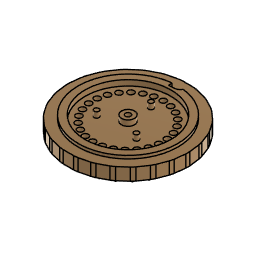
筐体 (Autodesk Fusion 360 archive; units mm, degrees)
design "ローターA"
Autodesk Fusion 360 part; units mm, degrees
sketch "スケッチ2" plane through (0, 0, 0) normal (0, 0, 1) x (1, 0, 0) in component "ローターA"
  circle A0 centre (0, 0) radius 23 construction
  circle A1 centre (0, 23) radius 2
  circle A2 centre (-5.5043, 22.3317) radius 2
  circle A3 centre (-10.6886, 20.3655) radius 2
  circle A4 centre (-15.2518, 17.2157) radius 2
  circle A5 centre (-18.9286, 13.0655) radius 2
  circle A6 centre (-21.5054, 8.1559) radius 2
  circle A7 centre (-22.8323, 2.7723) radius 2
  circle A8 centre (-22.8323, -2.7723) radius 2
  circle A9 centre (-21.5054, -8.1559) radius 2
  circle A10 centre (-18.9286, -13.0655) radius 2
  circle A11 centre (-15.2518, -17.2157) radius 2
  circle A12 centre (-10.6886, -20.3655) radius 2
  circle A13 centre (-5.5043, -22.3317) radius 2
  circle A14 centre (0, -23) radius 2
  circle A15 centre (5.5043, -22.3317) radius 2
  circle A16 centre (10.6886, -20.3655) radius 2
  circle A17 centre (15.2518, -17.2157) radius 2
  circle A18 centre (18.9286, -13.0655) radius 2
  circle A19 centre (21.5054, -8.1559) radius 2
  circle A20 centre (22.8323, -2.7723) radius 2
  circle A21 centre (22.8323, 2.7723) radius 2
  circle A22 centre (21.5054, 8.1559) radius 2
  circle A23 centre (18.9286, 13.0655) radius 2
  circle A24 centre (15.2518, 17.2157) radius 2
  circle A25 centre (10.6886, 20.3655) radius 2
  circle A26 centre (5.5043, 22.3317) radius 2
  circle A27 centre (0, 0) radius 4.25
  circle A28 centre (0, 0) radius 1.75
  circle A29 centre (0, 0) radius 28
  circle A30 centre (0, 0) radius 39
  line L0 (0, 0) -> (3.3913, -38.8523)
  line L1 (0, 0) -> (-3.3913, -38.8523)
  line L2 (3.3913, -38.8523) -> (-3.3913, -38.8523)
  line L3 (12.5907, -36.9117) -> (6.0052, -38.5349)
  line L4 (21.0584, -32.826) -> (15.0527, -35.978)
  line L5 (28.3022, -26.8325) -> (23.2254, -31.3302)
  line L6 (33.9013, -19.2796) -> (30.0483, -24.8616)
  line L7 (37.5301, -10.6063) -> (35.1249, -16.9481)
  line L8 (38.9778, -1.3165) -> (38.1602, -8.0497)
  line L9 (38.1602, 8.0497) -> (38.9778, 1.3165)
  line L10 (35.1249, 16.9481) -> (37.5301, 10.6063)
  line L11 (30.0483, 24.8616) -> (33.9013, 19.2796)
  line L12 (23.2254, 31.3302) -> (28.3022, 26.8325)
  line L13 (15.0527, 35.978) -> (21.0584, 32.826)
  line L14 (6.0052, 38.5349) -> (12.5907, 36.9117)
  line L15 (-3.3913, 38.8523) -> (3.3913, 38.8523)
  line L16 (-12.5907, 36.9117) -> (-6.0052, 38.5349)
  line L17 (-21.0584, 32.826) -> (-15.0527, 35.978)
  line L18 (-28.3022, 26.8325) -> (-23.2254, 31.3302)
  line L19 (-33.9013, 19.2796) -> (-30.0483, 24.8616)
  line L20 (-37.5301, 10.6063) -> (-35.1249, 16.9481)
  line L21 (-38.9778, 1.3165) -> (-38.1602, 8.0497)
  line L22 (-38.1602, -8.0497) -> (-38.9778, -1.3165)
  line L23 (-35.1249, -16.9481) -> (-37.5301, -10.6063)
  line L24 (-30.0483, -24.8616) -> (-33.9013, -19.2796)
  line L25 (-23.2254, -31.3302) -> (-28.3022, -26.8325)
  line L26 (-15.0527, -35.978) -> (-21.0584, -32.826)
  line L27 (-6.0052, -38.5349) -> (-12.5907, -36.9117)
  dimension "d10" = 46
  dimension "d11" = 4
  dimension "d13" = 360
  dimension "d24" = 8.5
  dimension "d37" = 3.5
  dimension "d64" = 56
  dimension "d65" = 78
  dimension "d67" = 360
  constraint coincident A0.centre A27.centre
  constraint coincident A0 A1.centre
  constraint concentric A0 A27
  constraint concentric A0 A28
  constraint concentric A0 A29
  constraint coincident A30 L0.end
  constraint coincident A30 L1.end
  constraint tangent A14 L0
  constraint tangent A14 L1
  measures "d10" diameter of A0
  measures "d11" diameter of A1
  measures "d24" diameter of A27
  measures "d37" diameter of A28
  measures "d64" diameter of A29
  measures "d65" diameter of A30
extrude "押し出し4" add sketch "スケッチ2" along normal blind 2 contours A14 A29 L0 L1 | A14 A27 L0 L1 | A27 A29 L0 L1 makes body 1 in component "ローターA"
sketch "スケッチ4" plane through (0, 0, 2) normal (0, 0, 1) x (-1, 0, 0) in component "ローターA"
  circle A0 centre (0, 0) radius 15 construction
  circle A1 centre (0, -15) radius 1.6
  circle A2 centre (12.9904, 7.5) radius 1.6
  circle A3 centre (-12.9904, 7.5) radius 1.6
  circle A4 centre (0, 0) radius 4.25
  circle A5 centre (-18.9286, -13.0655) radius 2
  circle A6 centre (-5.5043, -22.3317) radius 2
  circle A7 centre (-21.5054, -8.1559) radius 2
  circle A8 centre (15.2518, 17.2157) radius 2
  circle A9 centre (-10.6886, 20.3655) radius 2
  circle A10 centre (18.9286, 13.0655) radius 2
  circle A11 centre (10.6886, -20.3655) radius 2
  circle A12 centre (-15.2518, -17.2157) radius 2
  circle A13 centre (18.9286, -13.0655) radius 2
  circle A14 centre (-22.8323, 2.7723) radius 2
  circle A15 centre (-10.6886, -20.3655) radius 2
  circle A16 centre (-22.8323, -2.7723) radius 2
  circle A17 centre (21.5054, 8.1559) radius 2
  circle A18 centre (22.8323, -2.7723) radius 2
  circle A19 centre (15.2518, -17.2157) radius 2
  circle A20 centre (0, -23) radius 2
  circle A21 centre (22.8323, 2.7723) radius 2
  circle A22 centre (-5.5043, 22.3317) radius 2
  circle A23 centre (-18.9286, 13.0655) radius 2
  circle A24 centre (10.6886, 20.3655) radius 2
  circle A25 centre (-15.2518, 17.2157) radius 2
  circle A26 centre (-21.5054, 8.1559) radius 2
  circle A27 centre (5.5043, -22.3317) radius 2
  circle A28 centre (21.5054, -8.1559) radius 2
  circle A29 centre (5.5043, 22.3317) radius 2
  circle A30 centre (0, 23) radius 2
  circle A31 centre (0, 0) radius 28
  dimension "d31" = 30
  dimension "d32" = 3.2
  dimension "d16" = 3.2
  dimension "d17" = 3.2
  constraint coincident A0.centre A4.centre
  constraint coincident A0 A1.centre
  measures "d31" diameter of A0
  measures "d32" diameter of A1
  measures "d16" diameter of A3
  measures "d17" diameter of A2
extrude "押し出し8" add sketch "スケッチ4" along normal blind 8 contours A1 | A2 | A3 bodies 1 in component "ローターA"
extrude "押し出し9" add sketch "スケッチ2" along normal blind 10 contours A27 A28 L0 L1 | A27 A28 L0 L1 bodies 1 in component "ローターA"
extrude "押し出し13" add sketch "スケッチ2" along normal blind 8 contours A29 L0 L1 L2 | A29 A30 L0 L1 L3 L4 L5 L6 L7 L8 L9 L10 L11 L12 L13 L14 L15 L16 L17 L18 L19 L20 L21 L22 L23 L24 L25 L26 L27 bodies 1 in component "ローターA"
sketch "スケッチ9" plane through (0, 0, 0) normal (0, 0, 1) x (1, 0, 0) in component "ローターA"
  circle A0 centre (0, 0) radius 28
  circle A1 centre (18.9286, -13.0655) radius 2
  circle A2 centre (21.5054, -8.1559) radius 2
  circle A3 centre (22.8323, 2.7723) radius 2
  circle A4 centre (22.8323, -2.7723) radius 2
  circle A5 centre (21.5054, 8.1559) radius 2
  circle A6 centre (18.9286, 13.0655) radius 2
  circle A7 centre (15.2518, 17.2157) radius 2
  circle A8 centre (10.6886, 20.3655) radius 2
  circle A9 centre (5.5043, 22.3317) radius 2
  circle A10 centre (0, 23) radius 2
  circle A11 centre (-5.5043, 22.3317) radius 2
  circle A12 centre (-10.6886, 20.3655) radius 2
  circle A13 centre (-15.2518, 17.2157) radius 2
  circle A14 centre (-18.9286, 13.0655) radius 2
  circle A15 centre (-21.5054, 8.1559) radius 2
  circle A16 centre (-22.8323, 2.7723) radius 2
  circle A17 centre (-22.8323, -2.7723) radius 2
  circle A18 centre (-21.5054, -8.1559) radius 2
  circle A19 centre (-18.9286, -13.0655) radius 2
  circle A20 centre (-15.2518, -17.2157) radius 2
  circle A21 centre (-10.6886, -20.3655) radius 2
  circle A22 centre (-5.5043, -22.3317) radius 2
  circle A23 centre (0, -23) radius 2
  circle A24 centre (5.5043, -22.3317) radius 2
  circle A25 centre (10.6886, -20.3655) radius 2
  circle A26 centre (15.2518, -17.2157) radius 2
  circle A27 centre (0, 0) radius 30 construction
  circle A28 centre (0, 0) radius 34 construction
  circle A29 centre (0, 0) radius 32.5
  line L0 (-3.3413, 29.8133) -> (0, 0) construction
  arc A30 (0, 30) -> (-3.3413, 29.8133) centre (0, 0) ccw
  arc A31 (0, 30) -> (3.6197, 32.2978) centre (0, 34) ccw
  line L1 (-3.3413, 29.8133) -> (-3.6197, 32.2978)
  line L2 (-10.379, 28.1474) -> (-11.2439, 30.493)
  arc A32 (-7.1795, 29.1283) -> (-10.379, 28.1474) centre (0, 0) ccw
  arc A33 (-7.1795, 29.1283) -> (-4.2148, 32.2255) centre (-8.1367, 33.012) ccw
  line L3 (-16.8135, 24.8456) -> (-18.2147, 26.9161)
  arc A34 (-13.9417, 26.5637) -> (-16.8135, 24.8456) centre (0, 0) ccw
  arc A35 (-13.9417, 26.5637) -> (-11.8044, 30.2805) centre (-15.8006, 30.1055) ccw
  line L4 (-22.2709, 20.0999) -> (-24.1268, 21.7749)
  arc A36 (-19.8937, 22.4553) -> (-22.2709, 20.0999) centre (0, 0) ccw
  arc A37 (-19.8937, 22.4553) -> (-18.708, 26.5756) centre (-22.5462, 25.4494) ccw
  line L5 (-26.434, 14.1861) -> (-28.6368, 15.3683)
  arc A38 (-24.6895, 17.0419) -> (-26.434, 14.1861) centre (0, 0) ccw
  arc A39 (-24.6895, 17.0419) -> (-24.5243, 21.3262) centre (-27.9815, 19.3142) ccw
  line L6 (-29.0608, 7.4478) -> (-31.4825, 8.0684)
  arc A40 (-28.0505, 10.6381) -> (-29.0608, 7.4478) centre (0, 0) ccw
  arc A41 (-28.0505, 10.6381) -> (-28.9154, 14.8375) centre (-31.7906, 12.0566) ccw
  line L7 (-29.9987, 0.2767) -> (-32.4986, 0.2997)
  arc A42 (-29.7813, 3.6161) -> (-29.9987, 0.2767) centre (0, 0) ccw
  arc A43 (-29.7813, 3.6161) -> (-31.626, 7.4864) centre (-33.7521, 4.0982) ccw
  line L8 (-29.1932, -6.9105) -> (-31.626, -7.4864)
  arc A44 (-29.7813, -3.6161) -> (-29.1932, -6.9105) centre (0, 0) ccw
  arc A45 (-29.7813, -3.6161) -> (-32.4986, -0.2997) centre (-33.7521, -4.0982) ccw
  line L9 (-26.6911, -13.6961) -> (-28.9154, -14.8375)
  arc A46 (-28.0505, -10.6381) -> (-26.6911, -13.6961) centre (0, 0) ccw
  arc A47 (-28.0505, -10.6381) -> (-31.4825, -8.0684) centre (-31.7906, -12.0566) ccw
  line L10 (-22.6378, -19.6857) -> (-24.5243, -21.3262)
  arc A48 (-24.6895, -17.0419) -> (-22.6378, -19.6857) centre (0, 0) ccw
  arc A49 (-24.6895, -17.0419) -> (-28.6368, -15.3683) centre (-27.9815, -19.3142) ccw
  line L11 (-17.2689, -24.5313) -> (-18.708, -26.5756)
  arc A50 (-19.8937, -22.4553) -> (-17.2689, -24.5313) centre (0, 0) ccw
  arc A51 (-19.8937, -22.4553) -> (-24.1268, -21.7749) centre (-22.5462, -25.4494) ccw
  line L12 (-10.8964, -27.9512) -> (-11.8044, -30.2805)
  arc A52 (-13.9417, -26.5637) -> (-10.8964, -27.9512) centre (0, 0) ccw
  arc A53 (-13.9417, -26.5637) -> (-18.2147, -26.9161) centre (-15.8006, -30.1055) ccw
  line L13 (-3.8906, -29.7467) -> (-4.2148, -32.2255)
  arc A54 (-7.1795, -29.1283) -> (-3.8906, -29.7467) centre (0, 0) ccw
  arc A55 (-7.1795, -29.1283) -> (-11.2439, -30.493) centre (-8.1367, -33.012) ccw
  line L14 (3.3413, -29.8133) -> (3.6197, -32.2978)
  arc A56 (0, -30) -> (3.3413, -29.8133) centre (0, 0) ccw
  arc A57 (0, -30) -> (-3.6197, -32.2978) centre (0, -34) ccw
  line L15 (10.379, -28.1474) -> (11.2439, -30.493)
  arc A58 (7.1795, -29.1283) -> (10.379, -28.1474) centre (0, 0) ccw
  arc A59 (7.1795, -29.1283) -> (4.2148, -32.2255) centre (8.1367, -33.012) ccw
  line L16 (16.8135, -24.8456) -> (18.2147, -26.9161)
  arc A60 (13.9417, -26.5637) -> (16.8135, -24.8456) centre (0, 0) ccw
  arc A61 (13.9417, -26.5637) -> (11.8044, -30.2805) centre (15.8006, -30.1055) ccw
  line L17 (22.2709, -20.0999) -> (24.1268, -21.7749)
  arc A62 (19.8937, -22.4553) -> (22.2709, -20.0999) centre (0, 0) ccw
  arc A63 (19.8937, -22.4553) -> (18.708, -26.5756) centre (22.5462, -25.4494) ccw
  line L18 (26.434, -14.1861) -> (28.6368, -15.3683)
  arc A64 (24.6895, -17.0419) -> (26.434, -14.1861) centre (0, 0) ccw
  arc A65 (24.6895, -17.0419) -> (24.5243, -21.3262) centre (27.9815, -19.3142) ccw
  line L19 (29.0608, -7.4478) -> (31.4825, -8.0684)
  arc A66 (28.0505, -10.6381) -> (29.0608, -7.4478) centre (0, 0) ccw
  arc A67 (28.0505, -10.6381) -> (28.9154, -14.8375) centre (31.7906, -12.0566) ccw
  line L20 (29.9987, -0.2767) -> (32.4986, -0.2997)
  arc A68 (29.7813, -3.6161) -> (29.9987, -0.2767) centre (0, 0) ccw
  arc A69 (29.7813, -3.6161) -> (31.626, -7.4864) centre (33.7521, -4.0982) ccw
  line L21 (29.1932, 6.9105) -> (31.626, 7.4864)
  arc A70 (29.7813, 3.6161) -> (29.1932, 6.9105) centre (0, 0) ccw
  arc A71 (29.7813, 3.6161) -> (32.4986, 0.2997) centre (33.7521, 4.0982) ccw
  line L22 (26.6911, 13.6961) -> (28.9154, 14.8375)
  arc A72 (28.0505, 10.6381) -> (26.6911, 13.6961) centre (0, 0) ccw
  arc A73 (28.0505, 10.6381) -> (31.4825, 8.0684) centre (31.7906, 12.0566) ccw
  line L23 (22.6378, 19.6857) -> (24.5243, 21.3262)
  arc A74 (24.6895, 17.0419) -> (22.6378, 19.6857) centre (0, 0) ccw
  arc A75 (24.6895, 17.0419) -> (28.6368, 15.3683) centre (27.9815, 19.3142) ccw
  line L24 (17.2689, 24.5313) -> (18.708, 26.5756)
  arc A76 (19.8937, 22.4553) -> (17.2689, 24.5313) centre (0, 0) ccw
  arc A77 (19.8937, 22.4553) -> (24.1268, 21.7749) centre (22.5462, 25.4494) ccw
  line L25 (10.8964, 27.9512) -> (11.8044, 30.2805)
  arc A78 (13.9417, 26.5637) -> (10.8964, 27.9512) centre (0, 0) ccw
  arc A79 (13.9417, 26.5637) -> (18.2147, 26.9161) centre (15.8006, 30.1055) ccw
  line L26 (3.8906, 29.7467) -> (4.2148, 32.2255)
  arc A80 (7.1795, 29.1283) -> (3.8906, 29.7467) centre (0, 0) ccw
  arc A81 (7.1795, 29.1283) -> (11.2439, 30.493) centre (8.1367, 33.012) ccw
  circle A82 centre (0, 0) radius 1.75
  circle A83 centre (0, 0) radius 4.25
  circle A84 centre (0, 0) radius 18
  dimension "d70" = 56
  dimension "d71" = 60
  dimension "d72" = 68
  dimension "d73" = 65
  dimension "d74" = 4
  dimension "d76" = 360
  dimension "d79" = 36
  constraint coincident A28 A31.centre
  constraint tangent A27 A31
  constraint concentric A0 A29
  constraint coincident A0.centre A27.centre
  constraint coincident A27 A30.start
  constraint coincident A29 A31.end
  constraint coincident A29 L1.end
  constraint collinear L0 L1
  constraint concentric A76 A84
  measures "d70" diameter of A0
  measures "d71" diameter of A27
  measures "d72" diameter of A28
  measures "d73" diameter of A29
  measures "d74" radius of A31
  measures "d79" diameter of A84
extrude "押し出し14" add sketch "スケッチ9" against normal blind 5 contours A0 | A29 A30 A31 L1 L2 A32 A33 L3 A34 A35 L4 A36 A37 L5 A38 A39 L6 A40 A41 L7 A42 A43 L8 A44 A45 L9 A46 A47 L10 A48 A49 L11 A50 A51 L12 A52 A53 L13 A54 A55 L14 A56 A57 L15 A58 A59 L16 A60 A61 L17 A62 A63 L18 A64 A65 L19 A66 A67 L20 A68 A69 L21 A70 A71 L22 A72 A73 L23 A74 A75 L24 A76 A77 L25 A78 A79 L26 A80 A81 | A83 bodies 1 in component "ローターA"
copy_body "ボディ -> コンポーネント2" bodies 1 removing the originals makes body 2 in component "ローターA (1)"
extrude "押し出し1" add 1 faces at (-6.1521, -10.8292, 2) along direction (0, 0, 1) blind 4.4 on bodies 2 bodies 2 in component "ローターA (1)"
sketch "スケッチ1" plane through (0, 0, 8) normal (0, 0, 1) x (-1, 0, 0)
  arc A0 (0, -30) -> (-3.6197, -32.2978) centre (0, -34) ccw
  line L0 (3.3413, -29.8133) -> (3.6197, -32.2978)
  arc A1 (0, -30) -> (3.3413, -29.8133) centre (0, 0) ccw
  circle A2 centre (0, 0) radius 32.5
  circle A3 centre (0, 0) radius 28
  dimension "d9" = 56
  constraint concentric A2 A3
  measures "d9" diameter of A3
extrude "押し出し2" add sketch "スケッチ1" along normal blind 2 contours A0 L0 A1 A2 picked at (-5.9767, -30.17) bodies 2 in component "ローターA (1)"
component "ローターA" placed x (1, 0, 0) y (0, 1, 0) z (0, 0, 1) at (0, 0, 0)
component "ローターA (1)" placed x (1, 0, 0) y (0, 1, 0) z (0, 0, 1) at (0, 0, 0) in component "ローターA"
equation "d10 = ( 23 * 2 ) * 1 mm"
equation "d68 = 2.00 mm + 6 mm"
equation "d71 = d70 + 4 mm"
equation "d72 = d71 + 8 mm"
equation "d73 = d72 - 3 mm"
equation "d80 = 6.00 mm - 1.6 mm"

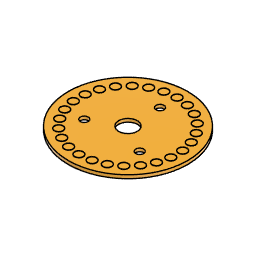
design "ローター基盤"
Autodesk Fusion 360 part; units mm, degrees
sketch "スケッチ1" plane through (0, 0, 0) normal (0, 0, 1) x (1, 0, 0)
  circle A0 centre (0, 0) radius 28
  circle A1 centre (0, 0) radius 23 construction
  circle A2 centre (0, 23) radius 2
  circle A3 centre (-5.5043, 22.3317) radius 2
  circle A4 centre (-10.6886, 20.3655) radius 2
  circle A5 centre (-15.2518, 17.2157) radius 2
  circle A6 centre (-18.9286, 13.0655) radius 2
  circle A7 centre (-21.5054, 8.1559) radius 2
  circle A8 centre (-22.8323, 2.7723) radius 2
  circle A9 centre (-22.8323, -2.7723) radius 2
  circle A10 centre (-21.5054, -8.1559) radius 2
  circle A11 centre (-18.9286, -13.0655) radius 2
  circle A12 centre (-15.2518, -17.2157) radius 2
  circle A13 centre (-10.6886, -20.3655) radius 2
  circle A14 centre (-5.5043, -22.3317) radius 2
  circle A15 centre (0, -23) radius 2
  circle A16 centre (5.5043, -22.3317) radius 2
  circle A17 centre (10.6886, -20.3655) radius 2
  circle A18 centre (15.2518, -17.2157) radius 2
  circle A19 centre (18.9286, -13.0655) radius 2
  circle A20 centre (21.5054, -8.1559) radius 2
  circle A21 centre (22.8323, -2.7723) radius 2
  circle A22 centre (22.8323, 2.7723) radius 2
  circle A23 centre (21.5054, 8.1559) radius 2
  circle A24 centre (18.9286, 13.0655) radius 2
  circle A25 centre (15.2518, 17.2157) radius 2
  circle A26 centre (10.6886, 20.3655) radius 2
  circle A27 centre (5.5043, 22.3317) radius 2
  dimension "d1" = 56
  dimension "d2" = 46
  dimension "d3" = 4
  dimension "d5" = 360
  constraint coincident A0.centre A1.centre
  constraint coincident A1 A2.centre
  measures "d1" diameter of A0
  measures "d2" diameter of A1
  measures "d3" diameter of A2
extrude "押し出し1" add sketch "スケッチ1" along normal blind 1.6 makes body 1
extrude "押し出し2" add sketch "スケッチ1" against normal blind 0.1 separate body contours A2 | A3 | A4 | A5 | A6 | A7 | A8 | A9 | A10 | A11 | A12 | A13 | A14 | A15 | A16 | A17 | A18 | A19 | A20 | A21 | A22 | A23 | A24 | A25 | A26 | A27 makes body 2 at (21.0897, -8.8759, 0) makes body 3 at (18.3138, 12.9661, 0) makes body 4 at (-11.0406, -19.27, 0) makes body 5 at (5.1709, 21.7543, 0) makes body 6 at (-5.4544, 21.7553, 0) makes body 7 at (-19.5435, -13.1649, 0) makes body 8 at (-23.248, -3.4923, 0) makes body 9 at (-23.4472, 2.673, 0) makes body 10 at (-10.0658, 19.9791, 0) makes body 11 at (15.8303, 17.2224, 0) makes body 12 at (15.7389, -18.4569, 0) makes body 13 at (0.0498, -23.5764, 0) makes body 14 at (22.2174, -2.8717, 0) makes body 15 at (21.0897, 7.436, 0) makes body 16 at (22.4166, 2.0524, 0) makes body 17 at (5.7478, -22.9522, 0) makes body 18 at (10.3367, 21.461, 0) makes body 19 at (-21.921, 7.436, 0) makes body 20 at (-15.4954, -16.5364, 0) makes body 21 at (-21.8165, -9.0291, 0) makes body 22 at (-19.3443, 12.3455, 0) makes body 23 at (-14.7631, 16.7623, 0) makes body 24 at (0.709, 23.5654, 0) makes body 25 at (18.513, -13.7854, 0) makes body 26 at (11.3115, -20.7519, 0) makes body 27 at (-5.2607, -22.9522, 0)
extrude "押し出し3" add sketch "スケッチ1" along normal blind 1.7 contours A2 | A3 | A4 | A5 | A6 | A7 | A8 | A9 | A10 | A11 | A12 | A13 | A14 | A15 | A16 | A17 | A18 | A19 | A20 | A21 | A22 | A23 | A24 | A25 | A26 | A27 bodies 1 2 3 4 5 6 7 8 9 10 11 12 13 14 15 16 17 18 19 20 21 22 23 24 25 26 27
sketch "スケッチ2" plane through (0, 0, 0) normal (0, 0, 1) x (1, 0, 0)
  circle A0 centre (0, 0) radius 15 construction
  circle A1 centre (0, 15) radius 2
  circle A2 centre (-12.9904, -7.5) radius 2
  circle A3 centre (12.9904, -7.5) radius 2
  circle A4 centre (0, 0) radius 4.5
  dimension "d12" = 30
  dimension "d13" = 4
  dimension "d15" = 360
  dimension "d16" = 9
  constraint coincident A0.centre A4.centre
  constraint coincident A0 A1.centre
  measures "d12" diameter of A0
  measures "d13" diameter of A1
  measures "d16" diameter of A4
extrude "押し出し4" cut sketch "スケッチ2" along normal up to surface (1.6 mm away) draft -5 bodies 1
copy_body "ボディ -> コンポーネント1" bodies 1 removing the originals makes body 28 in component "ローター基盤"
component "ローター基盤" placed x (1, 0, 0) y (0, 1, 0) z (0, 0, 1) at (0, 0, 0)
equation "d10 = 1.6 mm + 0.1 mm"

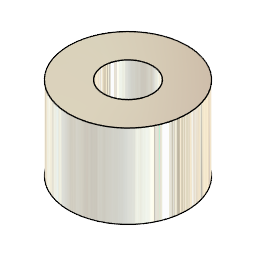
design "ロータースペーサー"
Autodesk Fusion 360 part; units mm, degrees
sketch "スケッチ1" plane through (0, 0, 0) normal (0, 0, 1) x (1, 0, 0)
  circle A0 centre (0, 0) radius 4.25
  circle A1 centre (0, 0) radius 1.75
  dimension "d1" = 3.5
  dimension "d2" = 8.5
  constraint coincident A0.centre A1.centre
  constraint concentric A0 A1
  measures "d1" diameter of A1
  measures "d2" diameter of A0
extrude "押し出し1" add sketch "スケッチ1" along normal blind 6 makes body 1
copy_body "ボディ -> コンポーネント1" bodies 1 removing the originals makes body 2 in component "ロータースペーサー"
component "ロータースペーサー" placed x (1, 0, 0) y (0, 1, 0) z (0, 0, 1) at (0, 0, 0)

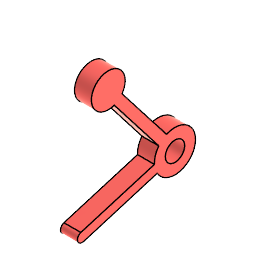
design "ラチェットストッパー"
Autodesk Fusion 360 part; units mm, degrees
sketch "スケッチ7" plane through (0, 0, 0) normal (1, 0, 0) x (0, 1, 0) in component "ラチェットストッパー 1"
  circle A0 centre (-13.9095, 17.7123) radius 3.5
  circle A1 centre (-0.1484, -0.0447) radius 2
  circle A2 centre (-0.1484, -0.0447) radius 2
  circle A3 centre (-0.1484, -0.0447) radius 4.25
  line L0 (-13.9095, 17.7123) -> (-0.1484, -0.0447) construction
  line L1 (-0.1129, -0.0906) -> (-13.9095, 17.7123) construction
  line L2 (-0.1484, -0.0447) -> (-19.2974, -5.8168) construction
  arc A4 (-19.5842, -4.8589) -> (-19.008, -6.7741) centre (-19.2974, -5.8168) ccw
  line L3 (-19.008, -6.7741) -> (-3.8251, -2.1765)
  line L4 (-0.1484, -0.0447) -> (-19.2974, -5.8168) construction
  line L5 (-1.8718, 0.4818) -> (-2.095, 0.4145)
  line L6 (-4.3918, -0.2818) -> (-19.5842, -4.8589)
  line L7 (-12.6841, 14.4338) -> (-3.4945, 2.5757)
  line L8 (-2.0168, 0.6689) -> (-1.8718, 0.4818)
  line L9 (-1.8847, 3.8344) -> (-11.0622, 15.6769)
  line L10 (-6.1824, -0.8212) -> (-5.6084, -2.7165)
  line L11 (-0.1484, -0.0447) -> (1.0781, -4.1139) construction
  dimension "d49" = 7
  dimension "d50" = 8.5
  dimension "d52" = 69
  dimension "d53" = 2
  dimension "d73" = 14
  dimension "d1" = 69
  dimension "d2" = 69
  dimension "d3" = 20
  constraint concentric A1 A2
  constraint concentric A2 A3
  constraint coincident A0.centre L0.start
  constraint coincident A1.centre A2.centre
  constraint parallel L0 L1
  constraint coincident L2.end A4.centre
  constraint parallel L2 L4
  constraint coincident A1 L5.end
  constraint coincident A3 L6.start
  constraint coincident A3 L7.end
  constraint coincident A1 L8.start
  constraint collinear L7 L8
  constraint coincident A3 L9.start
  constraint coincident A3 L3.end
  constraint coincident A0 L9.end
  constraint coincident A0 L7.start
  constraint coincident L6 L10.start
  constraint coincident L3 L10.end
  constraint perpendicular L3 L10
  constraint perpendicular L2 L11
  constraint coincident A3 L11.end
  measures "d49" diameter of A0
  measures "d50" diameter of A3
  measures "d52" angle of L1 L2
  measures "d53" diameter of A4
  measures "d73" distance of L2.end L10
  measures "d1" angle of L2 L7
  measures "d2" angle of L4 L9
  measures "d3" distance of A1.centre L2.end
extrude "押し出し1" add sketch "スケッチ7" along normal blind 3.5 in component "ラチェットストッパー"
component "ラチェットストッパー 1" placed x (1, 0, 0) y (0, 1, 0) z (0, 0, 1) at (0, 0, 0)
component "ラチェットストッパー" placed x (1, 0, 0) y (0, 1, 0) z (0, 0, 1) at (0, 0, 0) in component "ラチェットストッパー 1"
equation "d1 = d52"
equation "d2 = d52"

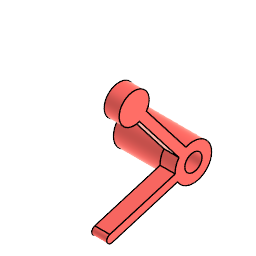
design "ラチェットストッパー&スペーサー"
Autodesk Fusion 360 part; units mm, degrees
sketch "スケッチ7" plane through (0, 0, 0) normal (1, 0, 0) x (0, 1, 0) in component "ラチェットストッパー 1"
  circle A0 centre (-13.9117, 17.7153) radius 3.5
  circle A1 centre (-0.1483, -0.0447) radius 2
  circle A2 centre (-0.1483, -0.0447) radius 2
  circle A3 centre (-0.1483, -0.0447) radius 4.25
  line L0 (-13.9117, 17.7153) -> (-0.1483, -0.0447) construction
  line L1 (-0.1124, -0.091) -> (-13.9117, 17.7153) construction
  line L2 (-0.1483, -0.0447) -> (-19.2973, -5.8168) construction
  arc A4 (-19.584, -4.8588) -> (-19.0078, -6.774) centre (-19.2973, -5.8168) ccw
  line L3 (-19.0078, -6.774) -> (-3.825, -2.1765)
  line L4 (-0.1483, -0.0447) -> (-19.2973, -5.8168) construction
  line L5 (-1.8713, 0.4819) -> (-2.0948, 0.4146)
  line L6 (-4.3917, -0.2817) -> (-19.584, -4.8588)
  line L7 (-12.686, 14.4369) -> (-3.4941, 2.5759)
  line L8 (-2.0165, 0.6693) -> (-1.8713, 0.4819)
  line L9 (-1.8848, 3.8344) -> (-11.0645, 15.6797)
  line L10 (-6.1822, -0.8212) -> (-5.6083, -2.7165)
  line L11 (-0.1483, -0.0447) -> (1.0783, -4.1139) construction
  dimension "d49" = 7
  dimension "d50" = 8.5
  dimension "d52" = 69
  dimension "d53" = 2
  dimension "d73" = 14
  dimension "d1" = 69
  dimension "d2" = 69
  dimension "d3" = 20
  constraint concentric A1 A2
  constraint concentric A2 A3
  constraint coincident A0.centre L0.start
  constraint coincident A1.centre A2.centre
  constraint parallel L0 L1
  constraint coincident L2.end A4.centre
  constraint parallel L2 L4
  constraint coincident A1 L5.end
  constraint coincident A3 L6.start
  constraint coincident A3 L7.end
  constraint coincident A1 L8.start
  constraint collinear L7 L8
  constraint coincident A3 L9.start
  constraint coincident A3 L3.end
  constraint coincident A0 L9.end
  constraint coincident A0 L7.start
  constraint coincident L6 L10.start
  constraint coincident L3 L10.end
  constraint perpendicular L3 L10
  constraint perpendicular L2 L11
  constraint coincident A3 L11.end
  measures "d49" diameter of A0
  measures "d50" diameter of A3
  measures "d52" angle of L1 L2
  measures "d53" diameter of A4
  measures "d73" distance of L2.end L10
  measures "d1" angle of L2 L7
  measures "d2" angle of L4 L9
  measures "d3" distance of A1.centre L2.end
extrude "押し出し1" add sketch "スケッチ7" along normal blind 3.5 in component "ラチェットストッパー"
sketch "スケッチ2" plane through (0, 0, 0) normal (-1, 0, 0) x (0, -1, 0)
  circle A0 centre (0.1483, -0.0447) radius 2
  line L0 (11.0645, 15.6797) -> (1.8848, 3.8344)
  arc A1 (1.8848, 3.8344) -> (3.825, -2.1765) centre (0.1483, -0.0447) ccw
  line L1 (3.825, -2.1765) -> (19.0078, -6.774)
  arc A2 (19.0078, -6.774) -> (19.584, -4.8588) centre (19.2973, -5.8168) ccw
  line L2 (19.584, -4.8588) -> (4.3917, -0.2817)
  arc A3 (4.3917, -0.2817) -> (3.4941, 2.5759) centre (0.1483, -0.0447) ccw
  line L3 (3.4941, 2.5759) -> (12.686, 14.4369)
  arc A4 (12.686, 14.4369) -> (11.0645, 15.6797) centre (13.9117, 17.7153) ccw
  circle A5 centre (0, 0) radius 4.25
  constraint coincident A5.centre origin
extrude "押し出し4" add sketch "スケッチ2" along normal blind 11 contours A1 A5 picked at (-3.1892, -1.0727) in component "ラチェットストッパー"
component "ラチェットストッパー 1" placed x (1, 0, 0) y (0, 1, 0) z (0, 0, 1) at (0, 0, 0)
component "ラチェットストッパー" placed x (1, 0, 0) y (0, 1, 0) z (0, 0, 1) at (0, 0, 0) in component "ラチェットストッパー 1"
equation "d1 = d52"
equation "d2 = d52"

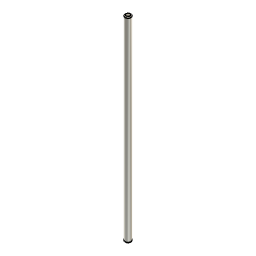
design "軸"
Autodesk Fusion 360 part; units mm, degrees
sketch "スケッチ1" plane through (0, 0, 0) normal (0, 0, 1) x (1, 0, 0)
  circle A0 centre (0, 0) radius 1.5
  dimension "d1" = 3
  constraint coincident A0.centre origin
  measures "d1" diameter of A0
extrude "押し出し1" add sketch "スケッチ1" along normal blind 100 makes body 1
copy_body "ボディ -> コンポーネント1" bodies 1 removing the originals makes body 2 in component "軸"
fillet "フィレット1" radius 0.5 2 edges at (-1.3985, -0.5424, 100) (-1.3985, -0.5424, 0) on bodies 2 in component "軸"
component "軸" placed x (1, 0, 0) y (0, 1, 0) z (0, 0, 1) at (0, 0, 0)
